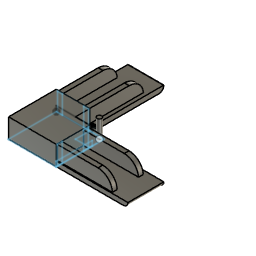
Screen Kit Corner (Autodesk Fusion 360 design; units mm, degrees)
Autodesk Fusion 360 part; units mm, degrees
sketch "Sketch1" plane through (0, 0, 0) normal (0, 0, 1) x (1, 0, 0)
  line L0 (-6.35, 6.35) -> (12.65, 6.35)
  line L1 (13.65, 5.35) -> (13.65, -13.65)
  line L2 (13.65, -13.65) -> (-6.35, -13.65)
  line L3 (-6.35, -13.65) -> (-6.35, 6.35)
  line L4 (13.65, 6.35) -> (7.65, 6.35)
  line L5 (7.65, 6.35) -> (7.65, 0.35)
  line L6 (7.65, 0.35) -> (13.65, 0.35)
  line L7 (13.65, 0.35) -> (13.65, 6.35)
  arc A0 (13.65, 5.35) -> (12.65, 6.35) centre (12.65, 5.35) ccw
  circle A1 centre (12.65, 5.35) radius 1
  dimension "d1" = 20
  dimension "d2" = 20
  dimension "d3" = 6
  dimension "d4" = 6
  dimension "d5" = 1
  dimension "d6" = 2
  constraint horizontal L0
  constraint vertical L1
  constraint horizontal L2
  constraint vertical L3
  constraint horizontal L4
  constraint vertical L5
  constraint horizontal L6
  constraint vertical L7
  constraint coincident L4.start L0
  constraint coincident L4.start L1
  constraint tangent L0 A0
  constraint tangent L1 A0
  constraint concentric A0 A1
  measures "d1" distance of L0.start L4.start
  measures "d2" distance of L0.start L2.end
  measures "d3" distance of L4.start L4.end
  measures "d4" distance of L4.start L6.end
  measures "d5" radius of A0
  measures "d6" diameter of A1
extrude "Extrude1" add sketch "Sketch1" along normal blind 8.1 contours L0 L1 L2 L3 L5 L6
extrude "Extrude2" add sketch "Sketch1" along normal blind 2.1 contours L0 L1 L4 L5 L6 L7 A1
extrude "Extrude3" add sketch "Sketch1" along normal blind 8 contours A0 A1
sketch "Sketch3" plane through (13.65, 0, 0) normal (1, 0, 0) x (0, 1, 0)
  line L0 (-13.65, 0) -> (5.35, 0)
  line L1 (5.35, 0) -> (5.35, 2.1)
  line L2 (5.35, 2.1) -> (0.35, 2.1)
  line L3 (0.35, 2.1) -> (0.35, 8.1)
  line L4 (0.35, 8.1) -> (-13.65, 8.1)
  line L5 (-13.65, 8.1) -> (-13.65, 0)
  line L6 (-13.208, 7.874) -> (-11.208, 7.874)
  line L7 (-11.208, 7.874) -> (-11.208, 0.0018)
  line L8 (-11.208, 0.0018) -> (-13.208, 0.0018)
  line L9 (-13.208, 0.0018) -> (-13.208, 7.874)
  line L10 (-0.254, 7.62) -> (-2.254, 7.62)
  line L11 (-2.254, 7.62) -> (-2.254, 0.0018)
  line L12 (-2.254, 0.0018) -> (-0.254, 0.0018)
  line L13 (-0.254, 0.0018) -> (-0.254, 7.62)
  dimension "d13" = 2
  dimension "d14" = 2
  constraint horizontal L6
  constraint vertical L7
  constraint horizontal L8
  constraint vertical L9
  constraint horizontal L10
  constraint vertical L11
  constraint horizontal L12
  constraint vertical L13
  measures "d13" distance of L6.start L6.end
  measures "d14" distance of L10.start L10.end
sketch "Sketch4" plane through (13.65, 0, 0) normal (1, 0, 0) x (0, 1, 0)
  line L0 (-13.6398, 0.0066) -> (1.3602, 0.0066)
  line L1 (1.3602, 0.0066) -> (1.3602, 2.0066)
  line L2 (1.3602, 2.0066) -> (-13.6398, 2.0066)
  line L3 (-13.6398, 2.0066) -> (-13.6398, 0.0066)
  dimension "d15" = 2
  dimension "d33" = 15
  constraint horizontal L0
  constraint vertical L1
  constraint horizontal L2
  constraint vertical L3
  measures "d15" distance of L0.start L2.end
  measures "d33" distance of L1.end L2.end
extrude "Extrude4" add sketch "Sketch4" along normal blind 30
extrude "Extrude5" add sketch "Sketch3" along normal blind 23 contours L0 L6 L7 L8 L9
sketch "Sketch5" plane through (13.65, 0, 0) normal (1, 0, 0) x (0, 1, 0)
extrude "Extrude6" add sketch "Sketch3" along normal blind 23 contours L0 L10 L11 L12 L13
fillet "Fillet1" radius 6 1 edges at (36.65, -12.208, 7.874)
fillet "Fillet2" radius 6 1 edges at (36.65, -1.254, 7.62)
fillet "Fillet3" radius 2 3 edges at (43.65, -6.1398, 0.0066) (43.65, -13.6398, 1.0066) (43.65, 1.3602, 1.0066)
sketch "Sketch6" plane through (0, 6.35, 0) normal (0, 1, 0) x (-1, 0, 0)
  line L0 (-12.65, 0) -> (6.35, 0)
  line L1 (6.35, 0) -> (6.35, 8.1)
  line L2 (6.35, 8.1) -> (-7.65, 8.1)
  line L3 (-7.65, 8.1) -> (-7.65, 2.1)
  line L4 (-7.65, 2.1) -> (-12.65, 2.1)
  line L5 (-12.65, 2.1) -> (-12.65, 0)
  line L6 (5.842, 7.62) -> (3.842, 7.62)
  line L7 (3.842, 7.62) -> (3.842, 0)
  line L8 (3.842, 0) -> (5.842, 0)
  line L9 (5.842, 0) -> (5.842, 7.62)
  line L10 (-7.112, 7.62) -> (-5.112, 7.62)
  line L11 (-5.112, 7.62) -> (-5.112, 0)
  line L12 (-5.112, 0) -> (-7.112, 0)
  line L13 (-7.112, 0) -> (-7.112, 7.62)
  line L14 (6.35, 0) -> (-8.65, 0)
  line L15 (-8.65, 0) -> (-8.65, 2.1)
  line L16 (-8.65, 2.1) -> (6.35, 2.1)
  line L17 (6.35, 2.1) -> (6.35, 0)
  dimension "d28" = 2
  dimension "d29" = 2
  dimension "d30" = 15
  constraint horizontal L6
  constraint vertical L7
  constraint horizontal L8
  constraint vertical L9
  constraint horizontal L10
  constraint vertical L11
  constraint horizontal L12
  constraint vertical L13
  constraint horizontal L14
  constraint vertical L15
  constraint horizontal L16
  constraint vertical L17
  constraint coincident L4 L15.end
  constraint coincident L0.end L1.start
  measures "d28" distance of L6.start L6.end
  measures "d29" distance of L10.start L10.end
  measures "d30" distance of L0.end L14.end
extrude "Extrude7" add sketch "Sketch6" along normal blind 30 contours L0 L4 L13 L14 L15 L16 | L0 L11 L12 L13 L14 L16 | L0 L7 L11 L14 L16 | L0 L7 L8 L9 L14 L16 | L0 L1 L9 L14 L16 L17
extrude "Extrude8" add sketch "Sketch6" along normal blind 23 contours L10 L11 L13 L16
extrude "Extrude9" add sketch "Sketch6" along normal blind 23 contours L6 L7 L9 L16
fillet "Fillet4" radius 6 1 edges at (6.112, 29.35, 7.62)
fillet "Fillet5" radius 6 1 edges at (-4.842, 29.35, 7.62)
fillet "Fillet6" radius 2 1 edges at (1.15, 36.35, 0)
